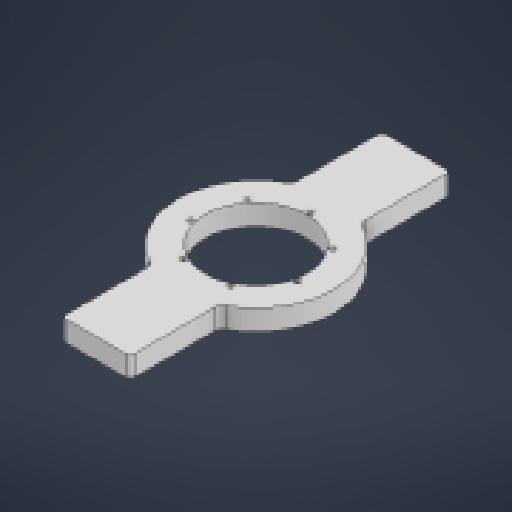
# Autodesk Inventor part: Head Thing
Saved by Autodesk Inventor 2025 (Build 290162000, 162)
## iProperties
Created: 2024-04-28
Part Number: Head Thing
Material: Generic
Document SubType Name: Modeling
Designer: Thienan Hoang
Density: 1 g/cm^3
Appearance: Default
Author: Thienan Hoang
Autodesk Inventor part; units mm, degrees
ref_plane "YZ Plane" through (0, 0, 0) normal (1, 0, 0) x (0, 1, 0)
ref_plane "XZ Plane" through (0, 0, 0) normal (0, 1, 0) x (-1, 0, 0)
ref_plane "XY Plane" through (0, 0, 0) normal (0, 0, 1) x (1, 0, 0)
sketch "Sketch1" plane through (0, 0, 0) normal (0, 1, 0) x (-1, 0, 0)
  circle A0 centre (0, 0) radius 37.5
  line L0 (25, 117.5) -> (-25, 117.5)
  line L1 (-25, -117.5) -> (25, -117.5)
  arc A1 (-25, 51.7808) -> (-25, -51.7808) centre (0, 0) ccw
  arc A2 (25, -51.7808) -> (25, 51.7808) centre (0, 0) ccw
  line L2 (-25, 117.5) -> (-25, 51.7808)
  line L3 (-25, -51.7808) -> (-25, -117.5)
  line L4 (25, -117.5) -> (25, -51.7808)
  line L5 (25, 51.7808) -> (25, 117.5)
  dimension "d0" = 75
  constraints: 12 end point, 5 parallel, 4 point on circle, 3 centre point, 2 coincident, 2 perpendicular, 1 horizontal
  measures "d0" diameter of A0
extrude "Extrusion1" add sketch "Sketch1" along normal blind 15
sketch "Sketch2" plane through (0, 15, 0) normal (0, 1, 0) x (1, 0, 0)
  circle A0 centre (0, 0) radius 40
  circle A1 centre (0, 40) radius 1.9
  circle A2 centre (-31.2733, 24.9396) radius 1.9
  circle A3 centre (-38.9971, -8.9008) radius 1.9
  circle A4 centre (-17.3553, -36.0388) radius 1.9
  circle A5 centre (17.3553, -36.0388) radius 1.9
  circle A6 centre (38.9971, -8.9008) radius 1.9
  circle A7 centre (31.2733, 24.9396) radius 1.9
  point P0 (-40, 0)
  point P1 (-24.9396, -31.2733)
  point P2 (8.9008, -38.9971)
  point P3 (36.0388, -17.3553)
  point P4 (36.0388, 17.3553)
  point P5 (8.9008, 38.9971)
  point P6 (-24.9396, 31.2733)
  dimension "d6" = 80
  dimension "d21" = 3.8
  dimension "d24" = 360
  constraints: 8 centre point, 2 point on circle, 1 coincident, 15 other
  measures "d6" diameter of A0
  measures "d21" diameter of A1
hole "Hole1" at (0, 15, -40) at (31.2733, 15, -24.9396) at (38.9971, 15, 8.9008) at (17.3553, 15, 36.0388) at (-17.3553, 15, 36.0388) at (-38.9971, 15, 8.9008) at (-31.2733, 15, -24.9396) direction (0, -1, 0) diameter 1.567 end through all thread size "M2x0.4" class "6H" standard "ANSI Metric M Profile"
extrude "Extrusion3" cut sketch "Sketch2" against normal blind 2 contours A7 A0 | A0 A7 | A6 A0 | A0 A6 | A1 A0 | A0 A1 | A5 A0 | A0 A5 | A2 A0 | A0 A2 | A4 A0 | A0 A4 | A3 A0 | A0 A3
fillet "Fillet1" radius 5 4 edges at (-25, 7.5, 51.7808) (25, 7.5, 51.7808) (25, 7.5, -51.7808) (-25, 7.5, -51.7808)
fillet "Fillet2" radius 3 4 edges at (25, 7.5, 117.5) (-25, 7.5, 117.5) (25, 7.5, -117.5) (-25, 7.5, -117.5)
chamfer "Chamfer1" distance 0.25 angle 45 34 edges at (25, 15, 84.6646) (25.6988, 15, 52.2798) (57.5, 15, 0) (25.6988, 15, -52.2798) (25, 15, -84.6646) (24.1213, 15, -116.6213) (0, 15, -117.5) (-24.1213, 15, -116.6213) (-25, 15, -84.6646) (-25.6988, 15, -52.2798) (-57.5, 15, 0) (-25.6988, 15, 52.2798) (-25, 15, 84.6646) (-24.1213, 15, 116.6213) (0, 15, 117.5) (24.1213, 15, 116.6213) (25, 0, 84.6646) (25.6988, 0, 52.2798) (57.5, 0, 0) (25.6988, 0, -52.2798) (25, 0, -84.6646) (24.1213, 0, -116.6213) (0, 0, -117.5) (-24.1213, 0, -116.6213) (-25, 0, -84.6646) (-25.6988, 0, -52.2798) (-57.5, 0, 0) (-25.6988, 0, 52.2798) (-25, 0, 84.6646) (-24.1213, 0, 116.6213) (0, 0, 117.5) (24.1213, 0, 116.6213) (37.5, 15, 0) (37.5, 0, 0)
body "Solid1"
